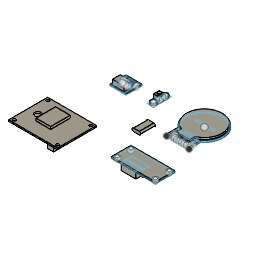
RoboClimeLib (Autodesk Fusion 360 design; units mm, degrees)
Autodesk Fusion 360 part; units mm, degrees
note: some values were not read from the file. Set by a fixed rule: which sketch regions a step uses.
sketch "Sketch1" plane through (0, 0, 0) normal (0, 0, 1) x (1, 0, 0)
  circle A0 centre (25, 25) radius 19
  circle A1 centre (25, 25) radius 18
  line L0 (36.5, 9.8755) -> (36.5, 0)
  line L1 (34.5, -2) -> (15.5, -2)
  line L2 (25, -2) -> (25, 6)
  line L3 (13.5, 0) -> (13.5, 9.8755)
  line L4 (15.5, -2) -> (13.5, 0)
  line L5 (36.5, 0) -> (34.5, -2)
  circle A2 centre (34.5, 4) radius 1
  circle A3 centre (15.5, 4) radius 1
  line L6 (17, 3) -> (32, 3)
  line L7 (18, 3) -> (18, 8.4169)
  line L8 (32, 3) -> (32, 8.4169)
  circle A4 centre (17.5, 0) radius 0.75
  circle A5 centre (20, 0) radius 0.75
  circle A6 centre (22.5, 0) radius 0.75
  circle A7 centre (25, 0) radius 0.75
  circle A8 centre (27.5, 0) radius 0.75
  circle A9 centre (30, 0) radius 0.75
  circle A10 centre (32.5, 0) radius 0.75
  line L9 (19.478, 11.9581) -> (31.478, 11.9581)
  line L10 (31.478, 11.9581) -> (31.478, 9.9581)
  line L11 (31.478, 9.9581) -> (19.478, 9.9581)
  line L12 (19.478, 9.9581) -> (19.478, 11.9581)
  line L13 (15, 28) -> (33, 28)
  line L14 (33, 28) -> (33, 26)
  line L15 (33, 26) -> (15, 26)
  line L16 (15, 26) -> (15, 28)
  point P0 (36.5, -2)
  point P1 (13.5, -2)
  dimension "d1" = 38
  dimension "d2" = 36
  dimension "d5" = 11.5
  dimension "d6" = 2
  dimension "d7" = 2
  dimension "d8" = 2
  dimension "d9" = 2
  dimension "d10" = 2
  dimension "d11" = 2
  dimension "d12" = 6
  dimension "d13" = 2
  dimension "d14" = 2
  dimension "d15" = 5
  dimension "d17" = 7
  dimension "d18" = 1.5
  dimension "d19" = 4
  dimension "d22" = 15
  dimension "d23" = 0
  dimension "d24" = 2
  dimension "d25" = 12
  dimension "d26" = 2
  constraint concentric A0 A1
  constraint vertical L0
  constraint horizontal L1
  constraint vertical L2
  constraint vertical L3
  constraint coincident L2.start L1
  constraint coincident A0 L0.start
  constraint coincident A0 L3.end
  constraint coincident A0 L2.end
  constraint coincident L1 P1
  constraint coincident P1 L3
  constraint coincident P0 L0
  constraint coincident P0 L1
  constraint horizontal L6
  constraint coincident L6 L7.start
  constraint perpendicular L6 L7
  constraint coincident A1 L8.end
  constraint coincident A1 L7.end
  constraint horizontal L9
  constraint vertical L10
  constraint horizontal L11
  constraint vertical L12
  constraint horizontal L13
  constraint vertical L14
  constraint horizontal L15
  constraint vertical L16
  measures "d1" diameter of A0
  measures "d2" diameter of A1
  measures "d5" distance of L2 L3
  measures "d6" distance of P1 L1.end
  measures "d7" distance of P1 L3.start
  measures "d8" distance of P0 L0.end
  measures "d9" distance of P0 L1.start
  measures "d10" diameter of A2
  measures "d11" distance of L0 A2.centre
  measures "d12" distance of L1 A2.centre
  measures "d13" diameter of A3
  measures "d14" distance of L3 A3.centre
  measures "d15" distance of L1 L6
  measures "d17" distance of L2 L7
  measures "d18" diameter of A4
  measures "d19" distance of L3 A4.centre
  measures "d24" distance of L9 L11
  measures "d25" distance of L10 L12
  measures "d26" distance of L13 L15
extrude "Extrude1" add sketch "Sketch1" along normal blind 3.5 contours A0 A1 L7 L8 | A0 L2 L6 L7 | A0 L2 L6 L8 | A1 | L9 L10 L11 L12 | L13 L14 L15 L16 picked at (18.7544, 7.7959) makes body 1
extrude "Extrude2" add sketch "Sketch1" along normal blind 3 separate body contours L2 A7 | L2 A7 | A4 | A5 | A6 | A8 | A9 | A10 makes body 2 at (22.1578, -0.6674, 2) makes body 3 at (33.2491, -0.0374, 2) makes body 4 at (25.7463, 0.0747, 2) makes body 5 at (19.6578, -0.6674, 2) makes body 6 at (29.6578, -0.6674, 2) makes body 7 at (27.1578, -0.6674, 2) makes body 8 at (17.1578, -0.6674, 2)
extrude "Extrude3" add sketch "Sketch1" along normal blind 1.8 contours A0 A1 L7 L8 | A0 L1 L2 L3 L4 L6 L7 A7 | A0 L0 L1 L2 L5 L6 L8 A7 picked at (7.2286, 29.3671) bodies 1 2 3 4 5 6 7 8
extrude "Extrude4" add sketch "Sketch1" against normal blind 1 contours L9 L10 L11 L12 | L13 L14 L15 L16 bodies 1
extrude "Extrude5" add sketch "Sketch1" against normal blind 1 contours L2 A7 | L2 A7 | A4 | A5 | A6 | A8 | A9 | A10 bodies 1
copy_body "Body->Comp1" bodies 1 removing the originals makes body 9 in component "DisplayTFT1-28"
sketch "Sketch2" plane through (0, 0, 0) normal (0, 0, 1) x (1, 0, 0)
  line L0 (-60, 30) -> (-43.7, 30)
  line L1 (-43.7, 30) -> (-43.7, 13.7)
  line L2 (-43.7, 13.7) -> (-60, 13.7)
  line L3 (-60, 13.7) -> (-60, 30)
  line L4 (-58, 14) -> (-46, 14)
  line L5 (-46, 14) -> (-46, 22)
  line L6 (-46, 22) -> (-58, 22)
  line L7 (-58, 22) -> (-58, 14)
  circle A0 centre (-45.7, 26) radius 1
  circle A1 centre (-58, 26) radius 1
  line L8 (-56, 29.0218) -> (-48, 29.0218)
  line L9 (-48, 29.0218) -> (-48, 27.5482)
  line L10 (-48, 27.5482) -> (-56, 27.5482)
  line L11 (-56, 27.5482) -> (-56, 29.0218)
  line L12 (-47, 22) -> (-48, 22)
  line L13 (-48, 22) -> (-48, 26.0003)
  line L14 (-48, 26.0003) -> (-47, 26.0003)
  line L15 (-47, 26.0003) -> (-47, 22)
  line L16 (-49.8333, 26.0003) -> (-49.8333, 22)
  line L17 (-50.8333, 26.0003) -> (-49.8333, 26.0003)
  line L18 (-50.8333, 22) -> (-50.8333, 26.0003)
  line L19 (-52.6667, 26.0003) -> (-52.6667, 22)
  line L20 (-53.6667, 26.0003) -> (-52.6667, 26.0003)
  line L21 (-53.6667, 22) -> (-53.6667, 26.0003)
  line L22 (-55.5, 26.0003) -> (-55.5, 22)
  line L23 (-56.5, 26.0003) -> (-55.5, 26.0003)
  line L24 (-56.5, 22) -> (-56.5, 26.0003)
  dimension "d37" = 16.3
  dimension "d38" = 16.3
  dimension "d39" = 12
  dimension "d40" = 8
  dimension "d41" = 2
  dimension "d42" = 4
  dimension "d43" = 2
  dimension "d44" = 2
  dimension "d45" = 2
  dimension "d46" = 4
  dimension "d55" = -8.5
  dimension "d56" = 0
  constraint horizontal L0
  constraint vertical L1
  constraint horizontal L2
  constraint vertical L3
  constraint horizontal L4
  constraint vertical L5
  constraint horizontal L6
  constraint vertical L7
  constraint horizontal L8
  constraint vertical L9
  constraint horizontal L10
  constraint vertical L11
  constraint horizontal L12
  constraint vertical L13
  constraint horizontal L14
  constraint vertical L15
  constraint coincident L6 L12.start
  measures "d37" distance of L0.start L0.end
  measures "d38" distance of L0.start L2.end
  measures "d39" distance of L4.start L4.end
  measures "d40" distance of L4.start L6.end
  measures "d41" diameter of A0
  measures "d42" distance of L0 A0.centre
  measures "d43" distance of L1 A0.centre
  measures "d44" diameter of A1
  measures "d45" distance of L3 A1.centre
  measures "d46" distance of L0 A1.centre
extrude "Extrude6" add sketch "Sketch2" along normal blind 6.4 separate body contours L4 L5 L6 L7 L12 makes body 10
extrude "Extrude7" add sketch "Sketch2" along normal blind 2.2 separate body contours L8 L9 L10 L11 makes body 11
extrude "Extrude8" add sketch "Sketch2" along normal blind 1.2 contours L0 L1 L2 L3 | L6 L22 L23 L24 | L6 L12 L13 L14 L15 | L6 L19 L20 L21 | L6 L16 L17 L18 bodies 10 11
extrude "Extrude9" add sketch "Sketch2" along normal blind 1.6 contours L6 L22 L23 L24 | L6 L12 L13 L14 L15 | L6 L19 L20 L21 | L6 L16 L17 L18 bodies 10
copy_body "Body->Comp2" bodies 10 removing the originals makes body 12 in component "SensorsModule"
sketch "Sketch3" plane through (0, 0, 0) normal (0, 0, 1) x (1, 0, 0)
  line L0 (-80, -30) -> (-30, -30)
  line L1 (-30, -30) -> (-30, -70)
  line L2 (-30, -70) -> (-80, -70)
  line L3 (-80, -70) -> (-80, -30)
  circle A0 centre (-77, -33) radius 1.5
  circle A1 centre (-33, -33) radius 1.5
  circle A2 centre (-77, -67) radius 1.5
  circle A3 centre (-33, -67) radius 1.5
  line L4 (-65, -37) -> (-50, -37)
  line L5 (-50, -37) -> (-50, -57)
  line L6 (-50, -57) -> (-65, -57)
  line L7 (-65, -57) -> (-65, -37)
  line L8 (-37, -35) -> (-43, -35)
  line L9 (-43, -35) -> (-43, -47.5)
  line L10 (-43, -47.5) -> (-37, -47.5)
  line L11 (-37, -47.5) -> (-37, -35)
  line L12 (-43, -52) -> (-37, -52)
  line L13 (-37, -52) -> (-37, -67)
  line L14 (-37, -67) -> (-43, -67)
  line L15 (-43, -67) -> (-43, -52)
  line L16 (-77, -53) -> (-71.0862, -53)
  line L17 (-71.0862, -53) -> (-71.0862, -61.0418)
  line L18 (-71.0862, -61.0418) -> (-77, -61.0418)
  line L19 (-77, -61.0418) -> (-77, -53)
  circle A4 centre (-70, -50) radius 3.2139
  dimension "d59" = 50
  dimension "d60" = 40
  dimension "d61" = 3
  dimension "d62" = 3
  dimension "d63" = 3
  dimension "d66" = 44
  dimension "d67" = -34
  dimension "d68" = 6
  dimension "d69" = 12.5
  dimension "d70" = 6
  dimension "d71" = 15
  constraint horizontal L0
  constraint vertical L1
  constraint horizontal L2
  constraint vertical L3
  constraint horizontal L4
  constraint vertical L5
  constraint horizontal L6
  constraint vertical L7
  constraint horizontal L8
  constraint vertical L9
  constraint horizontal L10
  constraint vertical L11
  constraint horizontal L12
  constraint vertical L13
  constraint horizontal L14
  constraint vertical L15
  constraint horizontal L16
  constraint vertical L17
  constraint horizontal L18
  constraint vertical L19
  measures "d59" distance of L0.start L0.end
  measures "d60" distance of L0.start L2.end
  measures "d61" diameter of A0
  measures "d62" distance of L3 A0.centre
  measures "d63" distance of L0 A0.centre
  measures "d68" distance of L8.start L8.end
  measures "d69" distance of L8.start L10.end
  measures "d70" distance of L12.start L12.end
  measures "d71" distance of L12.start L14.end
extrude "Extrude10" add sketch "Sketch3" along normal blind 1.5 separate body makes body 13
extrude "Extrude11" add sketch "Sketch3" along normal blind 4 contours L4 L5 L6 L7 bodies 13
extrude "Extrude12" add sketch "Sketch3" against normal blind 7 separate body contours L8 L9 L10 L11 | L12 L13 L14 L15 | L16 L17 L18 L19 A4 makes body 14 at (-37, -57, -2.3333) makes body 15 at (-37, -43.3333, -2.3333) makes body 16 at (-77, -58.3612, -2.3333)
extrude "Extrude13" add sketch "Sketch3" against normal blind 10 separate body contours L16 L17 A4 picked at (-69.7366, -48.957) makes body 17
fillet "Fillet1" radius 0.5 1 edges at (-68.8804, -46.9874, -10) on bodies 17
extrude "Extrude14" add sketch "Sketch3" along normal blind 1.5 contours L8 L9 L10 L11 | L12 L13 L14 L15 | L16 L17 L18 L19 A4 bodies 13 14 15 16 17
copy_body "Body->Comp3" bodies 13 removing the originals makes body 18 in component "MainBoard"
sketch "Sketch4" plane through (0, 0, 0) normal (0, 0, 1) x (1, 0, 0)
  line L0 (5, -30) -> (50, -30)
  line L1 (50, -30) -> (50, -50)
  line L2 (50, -50) -> (5, -50)
  line L3 (5, -50) -> (5, -30)
  circle A0 centre (8, -33) radius 1.5
  circle A1 centre (47, -33) radius 1.5
  circle A2 centre (8, -47) radius 1.5
  circle A3 centre (47, -47) radius 1.5
  line L4 (14, -49) -> (29, -49)
  line L5 (29, -49) -> (29, -43)
  line L6 (29, -43) -> (14, -43)
  line L7 (14, -43) -> (14, -49)
  line L8 (14, -38) -> (31.5, -38)
  line L9 (31.5, -38) -> (31.5, -44)
  line L10 (31.5, -44) -> (14, -44)
  line L11 (14, -44) -> (14, -38)
  dimension "d84" = 45
  dimension "d85" = 20
  dimension "d86" = 3
  dimension "d87" = 3
  dimension "d88" = 3
  dimension "d91" = 39
  dimension "d92" = -14
  dimension "d93" = 15
  dimension "d94" = 6
  dimension "d95" = 17.5
  dimension "d96" = 6
  constraint horizontal L0
  constraint vertical L1
  constraint horizontal L2
  constraint vertical L3
  constraint horizontal L4
  constraint vertical L5
  constraint horizontal L6
  constraint vertical L7
  constraint horizontal L8
  constraint vertical L9
  constraint horizontal L10
  constraint vertical L11
  measures "d84" distance of L0.start L0.end
  measures "d85" distance of L0.start L2.end
  measures "d86" diameter of A0
  measures "d87" distance of L0 A0.centre
  measures "d88" distance of L3 A0.centre
  measures "d93" distance of L4.start L4.end
  measures "d94" distance of L4.start L6.end
  measures "d95" distance of L8.start L8.end
  measures "d96" distance of L8.start L10.end
extrude "Extrude15" add sketch "Sketch4" against normal blind 7 separate body contours L4 L5 L7 L10 | L5 L6 L7 L10 L11 | L5 L6 L8 L9 L10 L11 makes body 19
extrude "Extrude16" add sketch "Sketch4" along normal blind 1.5 separate body makes body 20
extrude "Extrude17" add sketch "Sketch4" along normal blind 1.5 contours L4 L5 L7 L10 | L5 L6 L7 L10 L11 | L5 L6 L8 L9 L10 L11 bodies 19 20
copy_body "Body->Comp4" bodies 19 removing the originals makes body 21 in component "PowerBoard"
sketch "Sketch5" plane through (0, 0, 0) normal (0, 0, 1) x (1, 0, 0)
  line L0 (-25, 35) -> (-19, 35)
  line L1 (-19, 35) -> (-19, 17)
  line L2 (-19, 17) -> (-25, 17)
  line L3 (-25, 17) -> (-25, 35)
  line L4 (-25, 29) -> (-19, 29)
  line L5 (-25, 23) -> (-19, 23)
  circle A0 centre (-22, 26) radius 1.8
  circle A1 centre (-22, 20) radius 1.1
  circle A2 centre (-22, 32) radius 1.1
  dimension "d103" = 6
  dimension "d104" = 18
  dimension "d105" = 3.6
  dimension "d114" = 2.2
  dimension "d115" = 2.2
  constraint horizontal L0
  constraint vertical L1
  constraint horizontal L2
  constraint vertical L3
  constraint coincident L3 L4.start
  constraint coincident L1 L4.end
  constraint perpendicular L1 L4
  constraint coincident L3 L5.start
  constraint coincident L1 L5.end
  constraint perpendicular L1 L5
  measures "d103" distance of L0.start L0.end
  measures "d104" distance of L0.start L2.end
  measures "d105" diameter of A0
  measures "d114" diameter of A1
  measures "d115" diameter of A2
extrude "Extrude18" add sketch "Sketch5" along normal blind 6.5 separate body contours A0 makes body 22
extrude "Extrude19" add sketch "Sketch5" along normal blind 5.4 contours L1 L3 L4 L5 bodies 22
extrude "Extrude20" add sketch "Sketch5" along normal blind 1.5 contours L0 L1 L3 L4 | L1 L2 L3 L5 | A1 | A2 bodies 22
fillet "Fillet2" radius 0.25 1 edges at (-23.6782, 25.3491, 6.5) on bodies 22
extrude "Extrude21" cut sketch "Sketch5" along normal blind 7 contours A1 | A2 bodies 22
fillet "Fillet3" radius 3 4 edges at (-19, 17, 0.75) (-19, 35, 0.75) (-25, 17, 0.75) (-25, 35, 0.75) on bodies 22
chamfer "Chamfer1" distance 1 angle 45 2 edges at (-23.0256, 32.3978, 1.5) (-23.0256, 20.3978, 1.5) on bodies 22
copy_body "Body->Comp5" bodies 22 removing the originals makes body 23 in component "Key"
sketch "Sketch7" plane through (0, 0, 0) normal (0, 1, 0) x (1, 0, 0)
  line L0 (-1.5, -3) -> (-7.5, -3)
  line L1 (-9, -1.5) -> (-9, -1.3)
  line L2 (-7.5, 0.2) -> (-1.5, 0.2)
  line L3 (0, -1.3) -> (0, -1.5)
  arc A0 (-1.5, -3) -> (0, -1.5) centre (-1.5, -1.5) ccw
  arc A1 (0, -1.3) -> (-1.5, 0.2) centre (-1.5, -1.3) ccw
  arc A2 (-7.5, 0.2) -> (-9, -1.3) centre (-7.5, -1.3) ccw
  arc A3 (-9, -1.5) -> (-7.5, -3) centre (-7.5, -1.5) ccw
  point P0 (0, -3)
  point P1 (-9, -3)
  point P2 (0, 0.2)
  dimension "d121" = 9
  dimension "d122" = 3.2
  dimension "d123" = 1.5
  constraint horizontal L0
  constraint vertical L1
  constraint horizontal L2
  constraint vertical L3
  constraint coincident P0 L0
  constraint coincident P0 L3
  constraint tangent L0 A0
  constraint tangent L3 A0
  constraint coincident P2 L2
  constraint coincident P2 L3
  constraint tangent L2 A1
  constraint tangent L3 A1
  constraint equal A0 A1
  constraint tangent L1 A2
  constraint tangent L2 A2
  constraint equal A0 A2
  constraint coincident P1 L0
  constraint coincident P1 L1
  constraint tangent L0 A3
  constraint tangent L1 A3
  constraint equal A0 A3
  measures "d121" distance of P0 P1
  measures "d122" distance of P0 P2
  measures "d123" radius of A0
extrude "Extrude22" add sketch "Sketch7" against normal blind 15 separate body makes body 24
copy_body "Body->Comp6" bodies 24 removing the originals makes body 25 in component "USB-C"
component "DisplayTFT1-28" placed x (1, 0, 0) y (0, 1, 0) z (0, 0, 1) at (0, 0, 0)
component "SensorsModule" placed x (1, 0, 0) y (0, 1, 0) z (0, 0, 1) at (0, 0, 0)
component "MainBoard" placed x (1, 0, 0) y (0, 1, 0) z (0, 0, 1) at (0, 0, 0)
component "PowerBoard" placed x (1, 0, 0) y (0, 1, 0) z (0, 0, 1) at (0, 0, 0)
component "Key" placed x (1, 0, 0) y (0, 1, 0) z (0, 0, 1) at (0, 0, 0)
component "USB-C" placed x (1, 0, 0) y (0, 1, 0) z (0, 0, 1) at (0, 0, 0)
equation "d7 = d6"
equation "d9 = d8"
named bodies: "Key", "USB-C"
